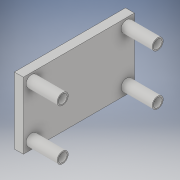
# Autodesk Inventor part: Part7
Saved by Autodesk Inventor 2019 (Build 230136000, 136)
## iProperties
Created: 2021-08-30
Part Number: Part7
Material: 一般
Document SubType Name: Sheet Metal
Designer: yuta
Density: 1 g/cm^3
Sheet Metal Rule: Default_mm
Appearance: 既定
Author: yuta
Autodesk Inventor part; units mm, degrees
ref_plane "YZ Plane" through (0, 0, 0) normal (1, 0, 0) x (0, 1, 0)
ref_plane "XZ Plane" through (0, 0, 0) normal (0, 1, 0) x (-1, 0, 0)
ref_plane "XY Plane" through (0, 0, 0) normal (0, 0, 1) x (1, 0, 0)
sketch "スケッチ1" plane through (0, 0, 0) normal (1, 0, 0) x (0, 1, 0)
  line L0 (13.9438, 85.4482) -> (-46.0562, 85.4482)
  line L1 (-46.0562, 85.4482) -> (-46.0562, -14.5518)
  line L2 (-46.0562, -14.5518) -> (13.9438, -14.5518)
  line L3 (13.9438, -14.5518) -> (13.9438, 85.4482)
  point P0 (0, 0)
  dimension "d0" = 60
  dimension "d1" = 100
  constraints: 8 end point, 2 parallel, 1 horizontal, 1 perpendicular
  measures "d0" distance of L2.end L1.end
  measures "d1" distance of L2.end L0.start
extrude "押し出し1" add sketch "スケッチ1" along normal blind 8.1
sketch "スケッチ2" plane through (8.1, 0, 0) normal (1, 0, 0) x (0, 0, -1)
  circle A0 centre (-78.096, 7.3739) radius 5
  circle A1 centre (-78.096, -38.2101) radius 5
  circle A2 centre (7.3739, -38.2101) radius 5
  circle A3 centre (7.3739, 7.3739) radius 5
  circle A4 centre (-78.096, 7.3739) radius 4
  circle A5 centre (-78.096, -38.2101) radius 4
  circle A6 centre (7.3739, 7.3739) radius 4
  circle A7 centre (7.3739, -38.2101) radius 4
  point P0 (0, 0)
  dimension "d4" = 10
  dimension "d5" = 10
  dimension "d6" = 10
  dimension "d7" = 10
  dimension "d8" = 8
  dimension "d9" = 8
  dimension "d10" = 8
  dimension "d11" = 8
  constraints: 8 centre point, 4 coincident
  measures "d4" diameter of A0
  measures "d5" diameter of A1
  measures "d6" diameter of A2
  measures "d7" diameter of A3
  measures "d8" diameter of A4
  measures "d9" diameter of A5
  measures "d10" diameter of A6
  measures "d11" diameter of A7
extrude "押し出し2" add sketch "スケッチ2" along normal blind 28
sketch "スケッチ3" plane through (0, 0, 0) normal (-1, 0, 0) x (0, 0, 1)
  point P0 (0, 0)
equation "\"BendRadius\" = Thickness"
equation "\"BendReliefWidth\" = Thickness"
equation "\"BendReliefDepth\" = 0.5 * Thickness"
equation "\"CornerReliefSize\" = 4 * Thickness"
equation "\"MinimumRemnant\" = 2 * Thickness"
equation "\"TransitionRadius\" = BendRadius"
equation "\"JacobiRadiusSize\" = BendRadius"
equation "\"GapSize\" = Thickness"
equation "\"Thickness\" = 0.5"
